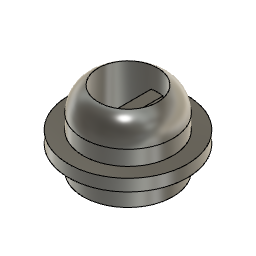
Landing_Shaft-LED-Top v3 (Autodesk Fusion 360 design; units mm, degrees)
Autodesk Fusion 360 part; units mm, degrees
sketch "Sketch1" plane through (0, 0, 0) normal (0, 0, 1) x (1, 0, 0)
  circle A0 centre (0, 0) radius 3.775
  circle A1 centre (0, 0) radius 1.5
  dimension "d1" = 7.55
  dimension "d2" = 3
  constraint coincident A0.centre A1.centre
  constraint concentric A0 A1
  measures "d1" diameter of A0
  measures "d2" diameter of A1
extrude "Extrude1" add sketch "Sketch1" along normal blind 5 makes body 1
fillet "Fillet1" radius 2.25 1 edges at (-3.5195, -1.3651, 5) on bodies 1
sketch "Sketch2" plane through (0, 0, 0) normal (0, 0, -1) x (1, 0, 0)
  circle A0 centre (0, 0) radius 1.5
  circle A1 centre (0, 0) radius 3.775
  circle A2 centre (0, 0) radius 2
  dimension "d7" = 4
  constraint concentric A0 A2
  measures "d7" diameter of A2
extrude "Extrude2" cut sketch "Sketch2" against normal blind 13.5 contours A2 bodies 1
extrude "Extrude3" cut 1 faces at (3.1618, -0.2869, 0) along direction (0, 0, 1) blind 1.5 on bodies 1 bodies 1
sketch "Sketch3" plane through (0, 0, 1.5) normal (0, 0, -1) x (1, 0, 0)
  circle A0 centre (0, 0) radius 2
  circle A1 centre (0, 0) radius 3.775
  circle A2 centre (0, 0) radius 5
  dimension "d12" = 10
  constraint concentric A0 A2
  measures "d12" diameter of A2
extrude "Extrude4" add sketch "Sketch3" along normal blind 1 separate body contours A2 makes body 2
extrude "Extrude5" add 1 faces at (3.1618, -0.2869, 1.5) along direction (0, 0, -1) blind 3 on bodies 1 bodies 1 2
sketch "Sketch4" plane through (0, 0, -1.5) normal (0, 0, -1) x (1, 0, 0)
  circle A0 centre (0, 0) radius 2
  circle A1 centre (0, 0) radius 3.775
  circle A2 centre (0, 0) radius 2.5
  dimension "d17" = 5
  constraint coincident A0.centre A1.centre
  measures "d17" diameter of A2
extrude "Extrude6" cut sketch "Sketch4" against normal blind 12.5 contours A2 bodies 1
sketch "Sketch5" plane through (0, 0, -1.5) normal (0, 0, -1) x (1, 0, 0)
  circle A0 centre (0, 0) radius 2.5
  circle A1 centre (0, 0) radius 3.775
  line L0 (0, 3.5) -> (0, -3.5) construction
  line L1 (0.5, 3.5) -> (0.5, -3.5)
  line L2 (-0.5, 3.5) -> (-0.5, -3.5)
  dimension "d20" = -0.5
  dimension "d21" = 0.5
  constraint vertical L0
extrude "Extrude7" add sketch "Sketch5" against normal blind 4.5 contours A0 L1 L2 bodies 1
